Autodesk Fusion 360 part; units mm, degrees
note: some values were not read from the file. Set by a fixed rule: which sketch regions a step uses.
(part 3 of 4)
  spline S124 degree 3 poles (20.1789, 42.1401) (19.8683, 42.9655) (19.3311, 43.6836) (18.669, 44.2614) (18.1917, 44.6778) (17.6457, 45.021) (17.0294, 45.2285) knots 0.1236 0.1236 0.1236 0.1236 0.632884 0.632884 0.632884 1 1 1 1
  spline S125 degree 3 poles (17.0294, 45.2285) (15.6679, 45.6868) (14.1945, 45.6326) (12.6935, 45.1125) (12.1298, 44.9172) (11.5566, 44.6602) (10.9624, 44.3448) knots 0 0 0 0 0.726997 0.726997 0.726997 1 1 1 1
  spline S126 degree 3 poles (10.9624, 44.3448) (10.8083, 44.263) (10.6793, 44.1929) (10.573, 44.1362) knots 0 0 0 0 0.122244 0.122244 0.122244 0.122244
  spline S127 degree 3 poles (10.573, 44.1362) (10.4946, 44.2052) (10.4022, 44.2872) (10.2936, 44.382) knots 0.893888 0.893888 0.893888 0.893888 1 1 1 1
  ellipse E6 centre (-1.4228, 24.3555) end of major axis (-10.8734, 2.8827) minor radius 14.2538 (10.2936, 44.382) -> (7.2449, 46.1286) ccw
  spline S128 degree 3 poles (7.2449, 46.1286) (6.4114, 46.403) (5.4613, 46.5014) (4.5483, 46.4889) (3.8849, 46.4798) (3.2641, 46.4203) (2.6738, 46.2166) knots 0.000001 0.000001 0.000001 0.000001 0.579134 0.579134 0.579134 1 1 1 1
  spline S129 degree 3 poles (2.6737, 46.2166) (0.624, 45.5094) (-0.7902, 43.8549) (-1.106, 41.9528) (-1.287, 40.8624) (-1.1003, 39.6959) (-0.5192, 38.6497) knots 0 0 0 0 0.618555 0.618555 0.618555 0.973163 0.973163 0.973163 0.973163
  spline S130 degree 3 poles (-0.5192, 38.6497) (-0.9554, 37.9197) (-1.2418, 37.1573) (-1.2576, 36.3503) (-1.2716, 35.6348) (-1.0747, 34.9439) (-0.7598, 34.2709) knots 0.006673 0.006673 0.006673 0.006673 0.533212 0.533212 0.533212 1 1 1 1
  spline S131 degree 3 poles (-0.7598, 34.2709) (0.1145, 32.4027) (1.9335, 31.179) (4.0147, 30.9406) knots 0 0 0 0 0.893312 0.893312 0.893312 0.893312
  spline S132 degree 3 poles (4.0147, 30.9406) (3.9761, 30.3012) (3.9008, 29.105) (3.8396, 28.1591) knots 0.081568 0.081568 0.081568 0.081568 1 1 1 1
  spline S133 degree 3 poles (29.7007, 2.1311) (29.5989, 2.131) (29.4934, 2.1308) (29.3841, 2.1308) knots 0.955909 0.955909 0.955909 0.955909 1 1 1 1
  spline S134 degree 3 poles (29.3841, 2.1308) (26.2893, 2.1292) (25.7344, 2.1938) (23.1155, 2.861) knots 0 0 0 0 1 1 1 1
  spline S135 degree 3 poles (23.1155, 2.861) (15.8271, 4.7179) (10.0738, 9.8891) (7.9282, 16.5117) knots 0 0 0 0 1 1 1 1
  spline S136 degree 3 poles (7.9282, 16.5117) (7.4178, 18.087) (7.2808, 18.6726) (7.0133, 20.4204) knots 0 0 0 0 1 1 1 1
  spline S137 degree 3 poles (7.0133, 20.4204) (6.814, 21.7234) (6.7809, 22.3775) (6.7737, 25.1631) knots 0 0 0 0 1 1 1 1
  spline S138 degree 3 poles (6.7737, 25.1631) (6.7643, 28.8189) (6.9545, 31.8997) (7.2227, 32.4341) knots 0 0 0 0 1 1 1 1
  spline S139 degree 3 poles (7.2227, 32.4341) (7.3731, 32.7338) (7.7563, 33.027) (8.0031, 33.0312) knots 0 0 0 0 1 1 1 1
  spline S140 degree 3 poles (8.0031, 33.0312) (8.0532, 33.032) (8.369, 32.8492) (8.705, 32.6248) knots 0 0 0 0 1 1 1 1
  spline S141 degree 3 poles (8.705, 32.6248) (9.2851, 32.2374) (9.8665, 32.0076) (11.2214, 31.6303) knots 0 0 0 0 1 1 1 1
  spline S142 degree 3 poles (11.2214, 31.6303) (11.8742, 31.4485) (11.8914, 31.4155) (11.7143, 30.6874) knots 0 0 0 0 1 1 1 1
  spline S143 degree 3 poles (11.7143, 30.6874) (10.9845, 27.6875) (10.9096, 23.7891) (11.5242, 20.7853) knots 0 0 0 0 1 1 1 1
  spline S144 degree 3 poles (11.5242, 20.7853) (12.8947, 14.087) (17.7674, 9.0084) (23.8364, 7.9527) knots 0 0 0 0 1 1 1 1
  spline S145 degree 3 poles (23.8364, 7.9527) (24.5674, 7.8255) (25.2101, 7.7982) (26.5177, 7.8388) knots 0 0 0 0 1 1 1 1
  spline S146 degree 3 poles (26.5177, 7.8388) (26.6332, 7.8424) (26.7451, 7.8465) (26.8538, 7.8512) knots 0 0 0 0 0.059413 0.059413 0.059413 0.059413
  spline S147 degree 3 poles (26.8538, 7.8512) (26.956, 7.4679) (27.0677, 7.0952) (27.1887, 6.732) (27.7682, 4.9924) (28.5742, 3.4395) (29.7007, 2.1311) knots 0.438432 0.438432 0.438432 0.438432 0.510571 0.510571 0.510571 0.856047 0.856047 0.856047 0.856047
  spline S148 degree 3 poles (26.6696, 28.6099) (26.7348, 28.5375) (26.8011, 28.467) (26.8689, 28.3977) (27.0173, 28.2462) (27.1722, 28.1018) (27.3333, 27.9647) (27.737, 27.6213) (28.176, 27.3243) (28.6406, 27.0754) knots 0.472088 0.472088 0.472088 0.472088 0.50252 0.50252 0.50252 0.569109 0.569109 0.569109 0.739021 0.739021 0.739021 0.739021
  spline S149 degree 3 poles (28.6406, 27.0754) (28.6443, 25.9855) (28.5938, 25.3432) (28.4946, 24.805) (28.467, 24.6548) (28.4349, 24.5095) (28.3963, 24.3575) (28.3479, 24.1671) (28.2888, 23.9667) (28.2121, 23.7367) knots 0.081283 0.081283 0.081283 0.081283 0.643747 0.643747 0.643747 0.800641 0.800641 0.800641 1 1 1 1
  spline S150 degree 3 poles (28.2121, 23.7367) (27.8013, 22.5041) (27.1671, 21.814) (26.6334, 21.506) (26.5949, 21.4839) (26.5569, 21.4635) (26.5191, 21.4448) knots 0 0 0 0 0.932819 0.932819 0.932819 1 1 1 1
  spline S151 degree 3 poles (26.5191, 21.4448) (26.1495, 21.2616) (26.0295, 21.2395) (26.0131, 21.2366) (26.0049, 21.2352) (26.0092, 21.2344) (25.9705, 21.2347) (25.9474, 21.235) (25.8975, 21.2362) (25.7646, 21.2632) knots 0.000002 0.000002 0.000002 0.000002 0.475564 0.475564 0.475564 0.711303 0.711303 0.711303 1 1 1 1
  spline S152 degree 3 poles (25.7646, 21.2632) (25.182, 21.3821) (24.7581, 21.6128) (24.2876, 22.1275) (24.0894, 22.3445) (23.8887, 22.6165) (23.6933, 22.956) (23.3548, 23.5442) (23.0502, 24.3309) (22.8535, 25.2998) knots 0 0 0 0 0.460583 0.460583 0.460583 0.654705 0.654705 0.654705 1 1 1 1
  spline S153 degree 3 poles (22.8535, 25.2998) (22.8074, 25.5265) (22.7339, 26.019) (22.6741, 26.5602) knots 0 0 0 0 0.263291 0.263291 0.263291 0.263291
  spline S154 degree 3 poles (22.6741, 26.5602) (22.7213, 26.5673) (22.7686, 26.5749) (22.8158, 26.583) (23.4027, 26.6834) (23.8706, 26.8599) (24.2061, 27.0017) knots 0.562128 0.562128 0.562128 0.562128 0.599835 0.599835 0.599835 1 1 1 1
  spline S155 degree 3 poles (24.2061, 27.0017) (25.082, 27.3721) (25.9389, 27.8878) (26.6696, 28.6099) knots 0.000003 0.000003 0.000003 0.000003 0.418346 0.418346 0.418346 0.418346
  spline S156 degree 3 poles (28.691, -3.3614) (32.9408, -3.4991) (36.8407, -2.8286) (40.1448, -1.2746) knots -0.538333 -0.538333 -0.538333 -0.538333 -0.206763 -0.206763 -0.206763 -0.206763
  spline S157 degree 3 poles (40.1448, -1.2746) (41.8108, -0.4911) (43.2001, 0.4189) (44.4435, 1.5947) knots 0 0 0 0 1 1 1 1
  spline S158 degree 3 poles (44.4435, 1.5947) (46.2822, 3.3334) (47.6676, 5.4847) (48.6623, 8.151) (48.7328, 8.34) (48.8016, 8.5317) (48.8687, 8.7262) (49.3481, 10.1146) (49.753, 11.6445) (50.1382, 13.3968) knots 0 0 0 0 0.632917 0.632917 0.632917 0.677783 0.677783 0.677783 1 1 1 1
  spline S159 degree 3 poles (50.1382, 13.3968) (51.1058, 17.7988) (51.5387, 21.0845) (51.8213, 26.4015) (51.8462, 26.8705) (51.8701, 27.3558) (51.8932, 27.8597) (51.8932, 27.8597) (51.8932, 27.8597) (51.8932, 27.8597) knots 0 0 0 0 0.918938 0.918938 0.918938 1 1 1 1.000001 1.000001 1.000001 1.000001
  spline S160 degree 3 poles (51.9001, 28.0088) (51.8978, 27.959) (51.8955, 27.9093) (51.8932, 27.8597) knots 1.612217 1.612217 1.612217 1.612217 1.675112 1.675112 1.675112 1.675112
  spline S161 degree 3 poles (51.9001, 28.0088) (53.1132, 28.4408) (54.2432, 29.0437) (55.2159, 29.8879) (55.4306, 30.0742) (55.637, 30.272) (55.8334, 30.481) (56.3444, 31.0248) (56.7853, 31.6466) (57.1251, 32.3371) knots 0.244983 0.244983 0.244983 0.244983 0.667487 0.667487 0.667487 0.760746 0.760746 0.760746 0.999997 0.999997 0.999997 0.999997
  spline S162 degree 3 poles (57.1251, 32.3371) (57.3415, 32.7769) (57.5858, 33.3542) (57.7015, 34.0837) (57.7667, 34.4952) (57.7814, 34.8692) (57.7845, 35.1895) (57.7846, 35.1948) (57.7846, 35.2002) (57.7847, 35.2056) knots 0.00001 0.00001 0.00001 0.00001 0.549059 0.549059 0.549059 0.90483 0.90483 0.90483 0.912062 0.912062 0.912062 0.912062
  line L17 (57.7847, 35.2056) -> (57.7832, 35.6708)
  spline S163 degree 3 poles (57.7832, 35.6708) (57.7831, 35.6767) (57.783, 35.6826) (57.7829, 35.6885) (57.7753, 36.1231) (57.7439, 36.6405) (57.6135, 37.201) (57.5259, 37.5777) (57.4101, 37.9108) (57.2954, 38.2005) knots 0.081345 0.081345 0.081345 0.081345 0.088946 0.088946 0.088946 0.543269 0.543269 0.543269 0.85612 0.85612 0.85612 0.85612
  spline S164 degree 3 poles (57.2954, 38.2005) (57.6289, 40.0462) (57.2005, 41.9011) (56.2368, 43.3879) (56.0215, 43.7199) (55.7793, 44.0349) (55.5119, 44.3297) (54.486, 45.4604) (53.1277, 46.2732) (51.6026, 46.6806) knots 0.058405 0.058405 0.058405 0.058405 0.508016 0.508016 0.508016 0.608426 0.608426 0.608426 1 1 1 1
  spline S165 degree 3 poles (51.6026, 46.6806) (50.3461, 47.0162) (49.0649, 46.9995) (47.8164, 46.7767) knots 0.000001 0.000001 0.000001 0.000001 0.638334 0.638334 0.638334 0.638334
  spline S166 degree 3 poles (47.8164, 46.7767) (47.5813, 47.0383) (47.3201, 47.2937) (47.0295, 47.534) (46.9498, 47.5999) (46.864, 47.6675) (46.7723, 47.7352) knots 0.700865 0.700865 0.700865 0.700865 0.939053 0.939053 0.939053 0.999998 0.999998 0.999998 0.999998
  spline S167 degree 3 poles (46.7723, 47.7352) (45.3302, 48.7994) (43.6443, 49.2146) (42.0523, 49.2386) (41.9141, 49.2407) (41.7762, 49.2398) (41.6389, 49.2361) (40.9851, 49.2182) (40.3133, 49.1301) (39.6411, 48.9493) knots 0.000002 0.000002 0.000002 0.000002 0.67158 0.67158 0.67158 0.729882 0.729882 0.729882 1 1 1 1
  spline S168 degree 3 poles (39.6411, 48.9493) (38.4909, 48.64) (37.4459, 48.1024) (36.5017, 47.4327) knots 0.000003 0.000003 0.000003 0.000003 0.699439 0.699439 0.699439 0.699439
  spline S169 degree 3 poles (36.5017, 47.4327) (34.5065, 48.0801) (32.3383, 47.9768) (30.4458, 47.0772) (28.9141, 46.3491) (27.639, 45.1486) (26.7459, 43.6578) knots 0.150615 0.150615 0.150615 0.150615 0.618328 0.618328 0.618328 1 1 1 1
  spline S170 degree 3 poles (26.7459, 43.6578) (26.4916, 43.2334) (26.2811, 42.7867) (26.1168, 42.3268) knots 0 0 0 0 0.168016 0.168016 0.168016 0.168016
  spline S171 degree 3 poles (26.1168, 42.3268) (25.625, 42.8719) (25.0259, 43.3578) (24.3244, 43.7251) (23.4812, 44.1666) (22.6044, 44.3989) (21.7478, 44.5189) knots 0.247509 0.247509 0.247509 0.247509 0.510228 0.510228 0.510228 0.845044 0.845044 0.845044 0.845044
  spline S172 degree 3 poles (21.7478, 44.5189) (21.336, 45.137) (20.8474, 45.6785) (20.3127, 46.145) (19.6364, 46.7352) (18.8102, 47.2669) (17.827, 47.5978) knots 0.340303 0.340303 0.340303 0.340303 0.632884 0.632884 0.632884 1 1 1 1
  spline S173 degree 3 poles (17.827, 47.5978) (15.8921, 48.2491) (13.8035, 48.1429) (11.8751, 47.4748) (11.5408, 47.359) (11.2106, 47.2283) (10.8834, 47.0845) knots 0 0 0 0 0.726997 0.726997 0.726997 0.855649 0.855649 0.855649 0.855649
  spline S174 degree 3 poles (10.8834, 47.0845) (10.0021, 47.6912) (9.04, 48.1696) (8.0266, 48.5032) knots 3.02631 3.02631 3.02631 3.02631 3.200385 3.200385 3.200385 3.200385
  spline S175 degree 3 poles (8.0266, 48.5032) (6.8258, 48.8985) (5.6304, 49.004) (4.514, 48.9887) (3.7224, 48.9778) (2.8175, 48.9108) (1.8584, 48.5799) knots 0.000001 0.000001 0.000001 0.000001 0.579134 0.579134 0.579134 1 1 1 1
  spline S176 degree 3 poles (1.8584, 48.5799) (-0.9926, 47.5963) (-3.0973, 45.223) (-3.5722, 42.3622) (-3.7722, 41.1577) (-3.6732, 39.9046) (-3.2719, 38.717) knots 0 0 0 0 0.618555 0.618555 0.618555 0.877662 0.877662 0.877662 0.877662
  spline S177 degree 3 poles (-3.2719, 38.717) (-3.5504, 38.0202) (-3.7407, 37.2387) (-3.7571, 36.3992) (-3.7807, 35.1938) (-3.4479, 34.1169) (-3.0241, 33.2113) knots 0.209942 0.209942 0.209942 0.209942 0.533212 0.533212 0.533212 1 1 1 1
  spline S178 degree 3 poles (-3.0241, 33.2113) (-2.118, 31.2751) (-0.5085, 29.8275) (1.3919, 29.0531) knots 0 0 0 0 0.64194 0.64194 0.64194 0.64194
  spline S179 degree 3 poles (1.3919, 29.0531) (1.3758, 28.8015) (1.3599, 28.5533) (1.3448, 28.3205) knots 0.773012 0.773012 0.773012 0.773012 1 1 1 1
  spline S180 degree 3 poles (1.3448, 28.3205) (1.1855, 25.8574) (1.2497, 22.768) (1.5259, 20.4573) knots 0 0 0 0 1 1 1 1
  spline S181 degree 3 poles (1.5259, 20.4573) (2.188, 14.9161) (4.3341, 9.9177) (7.8149, 5.9804) (8.3213, 5.4077) (8.8549, 4.8572) (9.4145, 4.3301) knots 2.814804 2.814804 2.814804 2.814804 3.195269 3.195269 3.195269 3.250613 3.250613 3.250613 3.250613
  spline S182 degree 3 poles (9.4145, 4.3301) (14.1533, -0.1335) (20.1834, -2.7036) (26.9457, -3.2616) (27.5221, -3.3091) (28.1039, -3.3424) (28.691, -3.3614) (28.691, -3.3614) (28.691, -3.3614) (28.691, -3.3614) knots 0 0 0 0 0.921454 0.921454 0.921454 1 1 1 1.000001 1.000001 1.000001 1.000001
  spline S183 degree 3 poles (28.8529, 1.636) (32.482, 1.5184) (35.5808, 2.1042) (38.0169, 3.25) knots -0.538331 -0.538331 -0.538331 -0.538331 -0.206759 -0.206759 -0.206759 -0.206759
  spline S184 degree 3 poles (38.0169, 3.25) (38.0169, 3.25) (38.0169, 3.25) (38.0169, 3.25) (39.3378, 3.8712) (40.1452, 4.4117) (41.0081, 5.2276) knots -0.000007 -0.000007 -0.000007 -0.000007 0 0 0 1 1 1 1
  spline S185 degree 3 poles (41.0081, 5.2276) (42.2991, 6.4485) (43.1918, 7.792) (43.9777, 9.8986) (44.0334, 10.048) (44.0883, 10.2011) (44.1425, 10.358) (44.5347, 11.4938) (44.8968, 12.8414) (45.2548, 14.4702) knots 0 0 0 0 0.632917 0.632917 0.632917 0.677783 0.677783 0.677783 1 1 1 1
  spline S186 degree 3 poles (45.2548, 14.4702) (46.1799, 18.6789) (46.5538, 21.5025) (46.8283, 26.6668) (46.8525, 27.1224) (46.8758, 27.5957) (46.8985, 28.0892) knots 0 0 0 0 0.918938 0.918938 0.918938 1 1 1 1
  spline S187 degree 3 poles (47.4971, 32.0539) (47.4947, 32.0505) (47.4924, 32.0471) (47.4902, 32.0437) (47.2657, 31.7128) (47.2344, 31.5681) (47.1957, 31.4563) (47.1118, 31.2144) (47.1097, 31.1501) (47.0977, 31.0856) (47.0666, 30.9194) (47.0663, 30.88) (47.06, 30.8195) (47.0394, 30.6238) (47.0264, 30.4292) (47.0081, 30.1441) (46.974, 29.6114) (46.9329, 28.8378) (46.8985, 28.0892) knots 0.02505 0.02505 0.02505 0.02505 0.025328 0.025328 0.025328 0.052584 0.052584 0.052584 0.111532 0.111532 0.111532 0.263489 0.263489 0.263489 0.755669 0.755669 0.755669 1.675088 1.675088 1.675088 1.675088
  spline S188 degree 3 poles (47.4971, 32.0539) (47.9897, 32.1595) (48.4824, 32.2652) (48.975, 32.3709) (50.3458, 32.665) (51.3246, 33.1312) (51.9386, 33.6641) (52.029, 33.7425) (52.1123, 33.8226) (52.1898, 33.9051) (52.3815, 34.1091) (52.5305, 34.3245) (52.6389, 34.5448) knots -0.155756 -0.155756 -0.155756 -0.155756 0.033409 0.033409 0.033409 0.667487 0.667487 0.667487 0.760746 0.760746 0.760746 0.999995 0.999995 0.999995 0.999995
  spline S189 degree 3 poles (52.6389, 34.5448) (52.6389, 34.5448) (52.6389, 34.5448) (52.6389, 34.5448) (52.7279, 34.7256) (52.7597, 34.8448) (52.7632, 34.8668) (52.7748, 34.9403) (52.7824, 35.0261) (52.7846, 35.2226) knots -0.000017 -0.000017 -0.000017 -0.000017 0 0 0 0.549059 0.549059 0.549059 0.896086 0.896086 0.896086 0.896086
  line L18 (52.7846, 35.2226) -> (52.7833, 35.6181)
  spline S190 degree 3 poles (52.7833, 35.6181) (52.7783, 35.8758) (52.7642, 35.9794) (52.7436, 36.0679) (52.7193, 36.1724) (52.6747, 36.3015) (52.5459, 36.602) knots 0.098297 0.098297 0.098297 0.098297 0.543269 0.543269 0.543269 1 1 1 1
  line L19 (52.5459, 36.602) -> (52.0202, 37.8281)
  line L20 (52.0202, 37.8281) -> (52.325, 38.8768)
  spline S191 degree 3 poles (52.325, 38.8768) (52.5054, 39.4971) (52.39, 40.1301) (52.0412, 40.6681) (51.9722, 40.7745) (51.8944, 40.8757) (51.8089, 40.97) (51.4582, 41.3565) (50.9527, 41.6789) (50.3122, 41.8499) knots 0.000001 0.000001 0.000001 0.000001 0.508016 0.508016 0.508016 0.608426 0.608426 0.608426 1 1 1 1
  spline S192 degree 3 poles (50.3122, 41.8499) (49.8357, 41.9772) (49.2359, 41.9882) (48.3226, 41.7781) (48.2236, 41.7553) (48.1214, 41.73) (48.016, 41.702) (47.8566, 41.6597) (47.6893, 41.6113) (47.5135, 41.5566) (46.8495, 41.3501) (46.1854, 41.1435) (45.5213, 40.937) knots 0 0 0 0 0.74388 0.74388 0.74388 0.824545 0.824545 0.824545 0.945665 0.945665 0.945665 1.335942 1.335942 1.335942 1.335942
  spline S193 degree 3 poles (45.5213, 40.937) (45.1993, 41.5534) (44.8773, 42.1698) (44.5552, 42.7862) (44.5311, 42.8323) (44.4975, 42.8908) (44.4575, 42.9537) (44.2603, 43.2641) (44.0459, 43.5132) (43.8431, 43.6809) (43.827, 43.6942) (43.8143, 43.704) (43.8035, 43.712) knots -0.495914 -0.495914 -0.495914 -0.495914 0.223295 0.223295 0.223295 0.361232 0.361232 0.361232 0.939053 0.939053 0.939053 1 1 1 1
  spline S194 degree 3 poles (43.8035, 43.712) (43.3808, 44.0239) (42.7445, 44.2276) (41.9768, 44.2392) (41.9102, 44.2402) (41.8429, 44.2398) (41.7751, 44.2379) (41.4784, 44.2298) (41.1969, 44.1901) (40.9398, 44.1209) knots 0.000002 0.000002 0.000002 0.000002 0.67158 0.67158 0.67158 0.729882 0.729882 0.729882 1 1 1 1
  spline S195 degree 3 poles (40.9397, 44.1209) (40.2839, 43.9445) (39.4481, 43.4741) (38.7124, 42.8035) knots 0.000001 0.000001 0.000001 0.000001 1 1 1 1
  line L21 (38.7124, 42.8035) -> (37.2495, 41.4699)
  spline S196 degree 3 poles (37.2495, 41.4699) (36.724, 41.767) (36.1986, 42.0641) (35.6731, 42.3611) (34.5938, 42.9714) (33.4845, 42.9855) (32.5924, 42.5614) (32.0115, 42.2853) (31.4617, 41.8003) (31.0351, 41.0882) knots -0.162297 -0.162297 -0.162297 -0.162297 0.019099 0.019099 0.019099 0.618328 0.618328 0.618328 1 1 1 1
  spline S197 degree 3 poles (31.0351, 41.0882) (30.7054, 40.5379) (30.5949, 39.9065) (30.737, 39.2208) (30.822, 38.8109) (30.9944, 38.3422) (31.2817, 37.8012) knots 0 0 0 0 0.647645 0.647645 0.647645 1 1 1 1
  line L22 (31.2817, 37.8012) -> (32.2313, 36.013)
  line L23 (32.2313, 36.013) -> (30.7684, 34.5336)
  spline S198 degree 3 poles (30.7684, 34.5336) (30.3425, 34.1029) (30.1555, 33.8199) (30.0718, 33.6163) (30.063, 33.595) (30.0551, 33.5742) (30.0479, 33.5532) (30.0006, 33.4158) (29.9666, 33.22) (29.9688, 32.9384) knots 0 0 0 0 0.54646 0.54646 0.54646 0.603605 0.603605 0.603605 1 1 1 1
  spline S199 degree 3 poles (29.9688, 32.9384) (29.9715, 32.5856) (30.1268, 32.2171) (30.4414, 31.8959) (30.4831, 31.8533) (30.5271, 31.8122) (30.5732, 31.7731) (30.8562, 31.5323) (31.2343, 31.3328) (31.6987, 31.2194) (32.2182, 31.0926) (32.7376, 30.9658) (33.2571, 30.839) knots 0 0 0 0 0.50252 0.50252 0.50252 0.569109 0.569109 0.569109 0.954182 0.954182 0.954182 1.198713 1.198713 1.198713 1.198713
  spline S200 degree 3 poles (33.6349, 27.6578) (33.6265, 28.1881) (33.6121, 28.719) (33.5943, 29.1314) (33.5834, 29.3845) (33.5734, 29.5797) (33.5545, 29.7812) (33.5487, 29.8427) (33.5428, 29.9038) (33.5287, 29.9983) (33.5177, 30.0719) (33.5151, 30.1431) (33.445, 30.3784) (33.4163, 30.4747) (33.3945, 30.5926) (33.2571, 30.839) knots -1.60234 -1.60234 -1.60234 -1.60234 -0.832399 -0.832399 -0.832399 -0.359926 -0.359926 -0.359926 -0.215638 -0.215638 -0.215638 -0.103142 -0.103142 -0.103142 -0.0571 -0.0571 -0.0571 -0.0571
  spline S201 degree 3 poles (33.6349, 27.6578) (33.6595, 26.1101) (33.6111, 24.9803) (33.4119, 23.899) (33.3633, 23.6355) (33.3064, 23.3782) (33.2423, 23.126) (33.1601, 22.8028) (33.0643, 22.4819) (32.9556, 22.1557) knots 0.000004 0.000004 0.000004 0.000004 0.643747 0.643747 0.643747 0.800641 0.800641 0.800641 1 1 1 1
  spline S202 degree 3 poles (32.9556, 22.1557) (32.2317, 19.9839) (30.9202, 18.2069) (29.1322, 17.1752) (29.0034, 17.1009) (28.8723, 17.0307) (28.7391, 16.9647) knots 0 0 0 0 0.932819 0.932819 0.932819 1 1 1 1
  spline S203 degree 3 poles (28.7391, 16.9647) (28.1265, 16.6611) (27.5201, 16.4228) (26.8636, 16.3095) (26.5381, 16.2533) (26.2135, 16.2321) (25.9203, 16.235) (25.5368, 16.2389) (25.1482, 16.286) (24.7656, 16.3641) knots 0 0 0 0 0.475564 0.475564 0.475564 0.711303 0.711303 0.711303 1 1 1 1
  spline S204 degree 3 poles (24.7656, 16.3641) (23.1787, 16.6877) (21.7086, 17.538) (20.5969, 18.7544) (20.1283, 19.2671) (19.7176, 19.8402) (19.3597, 20.4621) (18.714, 21.584) (18.2438, 22.8744) (17.9534, 24.3051) knots 0 0 0 0 0.460583 0.460583 0.460583 0.654705 0.654705 0.654705 1 1 1 1
  spline S205 degree 3 poles (17.9534, 24.3051) (17.831, 24.9081) (17.7431, 25.6067) (17.667, 26.3655) (17.6316, 26.7176) (17.6007, 27.0766) (17.5759, 27.4273) (17.5378, 27.9642) (17.5129, 28.4767) (17.5049, 28.924) (17.4937, 29.549) (17.4825, 30.174) (17.4713, 30.7991) knots 0 0 0 0 0.312333 0.312333 0.312333 0.457255 0.457255 0.457255 0.680586 0.680586 0.680586 1.042282 1.042282 1.042282 1.042282
  spline S206 degree 3 poles (20.5802, 31.4721) (20.0763, 31.4736) (19.6513, 31.4671) (19.2861, 31.444) (19.1179, 31.4334) (18.9789, 31.4265) (18.7326, 31.3824) (18.6233, 31.3629) (18.5023, 31.3481) (18.2322, 31.2466) (18.1014, 31.1975) (17.9317, 31.1353) (17.6625, 30.947) (17.6036, 30.9057) (17.5377, 30.858) (17.4713, 30.7991) knots 2.063963 2.063963 2.063963 2.063963 2.635195 2.635195 2.635195 2.89832 2.89832 2.89832 3.015054 3.015054 3.015054 3.071597 3.071597 3.071597 3.08397 3.08397 3.08397 3.08397
  spline S207 degree 3 poles (20.5802, 31.4721) (21.2817, 31.47) (21.6536, 31.4748) (21.8409, 31.4937) (21.891, 31.4987) (21.9311, 31.5042) (21.9723, 31.5113) (22.0174, 31.519) (22.1165, 31.5468) (22.259, 31.6071) (22.259, 31.6071) (22.259, 31.6071) (22.2591, 31.6071) knots 0 0 0 0 0.47317 0.47317 0.47317 0.599835 0.599835 0.599835 1 1 1 1.00001 1.00001 1.00001 1.00001
  spline S208 degree 3 poles (22.2591, 31.6071) (22.8153, 31.8423) (23.1441, 32.116) (23.3079, 32.3433) (23.3351, 32.381) (23.3587, 32.4182) (23.3798, 32.4562) (23.4541, 32.5898) (23.5115, 32.7711) (23.5276, 32.9724) knots 0.000003 0.000003 0.000003 0.000003 0.559796 0.559796 0.559796 0.65253 0.65253 0.65253 1 1 1 1
  spline S209 degree 3 poles (23.5276, 32.9724) (23.5484, 33.2315) (23.5378, 33.2897) (23.536, 33.2991) (23.5329, 33.3147) (23.5221, 33.3646) (23.4326, 33.5601) (23.4326, 33.5601) (23.4326, 33.5602) (23.4326, 33.5602) knots 0 0 0 0 0.532706 0.532706 0.532706 1 1 1 1.00001 1.00001 1.00001 1.00001
  spline S210 degree 3 poles (23.4326, 33.5602) (23.2318, 33.9987) (22.7513, 34.604) (21.9766, 35.1834) knots 0.355118 0.355118 0.355118 0.355118 0.81789 0.81789 0.81789 0.81789
  spline S211 degree 3 poles (21.9766, 35.1834) (22.2344, 35.7237) (22.4922, 36.2639) (22.75, 36.8042) (22.821, 36.9529) (22.8776, 37.1492) (22.8965, 37.372) (22.9021, 37.4387) (22.907, 37.5155) (22.9112, 37.6065) knots -0.861715 -0.861715 -0.861715 -0.861715 0.077995 0.077995 0.077995 0.83962 0.83962 0.83962 1 1 1 1
  spline S212 degree 3 poles (22.9112, 37.6065) (22.9267, 37.9446) (22.9226, 38.029) (22.9163, 38.0717) (22.9157, 38.076) (22.915, 38.0803) (22.9141, 38.0851) knots 0 0 0 0 0.440308 0.440308 0.440308 0.484514 0.484514 0.484514 0.484514
  spline S213 degree 3 poles (22.9141, 38.0851) (22.9136, 38.0875) (22.9006, 38.1464) (22.8052, 38.3453) (22.7894, 38.3781) (22.7719, 38.414) (22.7524, 38.4537) knots 0.500669 0.500669 0.500669 0.500669 0.930484 0.930484 0.930484 1 1 1 1
  spline S214 degree 3 poles (22.7524, 38.4537) (22.5414, 38.8823) (22.2676, 39.1581) (22.0052, 39.2955) (21.7005, 39.455) (21.2598, 39.5735) (20.5069, 39.6207) (20.4537, 39.6241) (20.3992, 39.627) (20.3434, 39.6297) knots 0 0 0 0 0.510228 0.510228 0.510228 0.967706 0.967706 0.967706 1 1 1 1
  line L24 (20.3434, 39.6297) -> (18.4188, 39.7197)
  spline S215 degree 3 poles (18.4188, 39.7197) (18.2256, 40.2329) (18.0324, 40.7461) (17.8392, 41.2593) (17.6948, 41.643) (17.4188, 42.0343) (17.0253, 42.3777) (16.7471, 42.6205) (16.4812, 42.7752) (16.2319, 42.8591) knots -0.193067 -0.193067 -0.193067 -0.193067 0.1236 0.1236 0.1236 0.632884 0.632884 0.632884 1 1 1 1
  spline S216 degree 3 poles (16.2319, 42.8591) (15.4436, 43.1244) (14.5856, 43.1223) (13.5119, 42.7503) (13.0939, 42.6055) (12.6374, 42.4036) (12.1347, 42.1367) knots 0 0 0 0 0.726997 0.726997 0.726997 1 1 1 1
  spline S217 degree 3 poles (12.1347, 42.1367) (11.9925, 42.0612) (11.8697, 41.9944) (11.7497, 41.9304) (11.2403, 41.6587) (10.731, 41.387) (10.2217, 41.1153) knots 0 0 0 0 0.122244 0.122244 0.122244 0.708101 0.708101 0.708101 0.708101
  spline S218 degree 3 poles (10.2217, 41.1153) (9.7883, 41.4966) (9.3549, 41.878) (8.9216, 42.2593) (8.8359, 42.3347) (8.749, 42.4119) (8.6504, 42.4979) knots 0.307309 0.307309 0.307309 0.307309 0.893888 0.893888 0.893888 1 1 1 1
  spline S219 degree 3 poles (8.6504, 42.4979) (7.9831, 43.0799) (7.2588, 43.492) (6.4631, 43.754) knots 2.954129 2.954129 2.954129 2.954129 3.200387 3.200387 3.200387 3.200387
  spline S220 degree 3 poles (6.4631, 43.754) (5.9969, 43.9074) (5.2921, 43.9989) (4.5826, 43.9891) (4.0473, 43.9818) (3.7108, 43.9298) (3.4891, 43.8533) knots 0.000001 0.000001 0.000001 0.000001 0.579134 0.579134 0.579134 1 1 1 1
  spline S221 degree 3 poles (3.4891, 43.8533) (2.2407, 43.4226) (1.5169, 42.4869) (1.3603, 41.5434) (1.2719, 41.011) (1.3578, 40.4189) (1.6662, 39.8637) (1.8994, 39.4439) (2.1326, 39.0241) (2.3658, 38.6043) knots 0.000001 0.000001 0.000001 0.000001 0.618555 0.618555 0.618555 0.973163 0.973163 0.973163 1.115459 1.115459 1.115459 1.115459
  spline S222 degree 3 poles (2.3658, 38.6043) (2.1195, 38.1921) (1.8732, 37.7798) (1.6269, 37.3676) (1.3366, 36.8816) (1.2467, 36.548) (1.2419, 36.3014) (1.2375, 36.0758) (1.2985, 35.771) (1.5046, 35.3306) knots -0.290647 -0.290647 -0.290647 -0.290647 0.006673 0.006673 0.006673 0.533212 0.533212 0.533212 1 1 1 1
  spline S223 degree 3 poles (1.5046, 35.3306) (1.9464, 34.3864) (2.8224, 33.7143) (3.9435, 33.4815) (4.0598, 33.4573) (4.1785, 33.4382) (4.2992, 33.4244) (5.0838, 33.3345) (5.8684, 33.2446) (6.653, 33.1547) knots 0 0 0 0 0.809326 0.809326 0.809326 0.893312 0.893312 0.893312 1.230091 1.230091 1.230091 1.230091
  spline S224 degree 3 poles (6.653, 33.1547) (6.6054, 32.3665) (6.5578, 31.5782) (6.5101, 30.7899) (6.471, 30.1427) (6.3958, 28.9474) (6.3344, 27.9977) knots -1.050718 -1.050718 -1.050718 -1.050718 0.081568 0.081568 0.081568 1 1 1 1
  spline S225 degree 3 poles (6.3344, 27.9977) (6.2001, 25.9217) (6.2704, 22.8924) (6.4905, 21.0506) knots 0 0 0 0 1 1 1 1
  spline S226 degree 3 poles (6.4905, 21.0506) (7.1275, 15.7208) (9.3016, 11.3051) (12.8428, 7.9698) knots 2.814805 2.814805 2.814805 2.814805 3.250616 3.250616 3.250616 3.250616
  spline S227 degree 3 poles (12.8428, 7.9698) (12.8428, 7.9698) (12.8428, 7.9698) (12.8428, 7.9698) (16.7533, 4.2864) (21.585, 2.1977) (27.3568, 1.7215) (27.8488, 1.6809) (28.3475, 1.6523) (28.8529, 1.636) knots -0.000002 -0.000002 -0.000002 -0.000002 0 0 0 0.921454 0.921454 0.921454 1 1 1 1
  dimension "d24" = 2.5
  dimension "d25" = -2.5
sketch "Sketch4" plane through (0, 0, -2) normal (0, 0, -1) x (1, 0, 0)
  spline S0 degree 3 poles (26.0631, 15.8423) (26.0024, 13.4447) (26.1457, 11.3703) (26.4797, 9.5307) knots 0.017136 0.017136 0.017136 0.017136 0.337125 0.337125 0.337125 0.337125
  spline S1 degree 3 poles (26.4797, 9.5307) (25.4741, 9.5023) (24.427, 9.5799) (23.6217, 9.7658) knots 0.450431 0.450431 0.450431 0.450431 1 1 1 1
  spline S2 degree 3 poles (23.6217, 9.7658) (21.0994, 10.3485) (19.0072, 11.5487) (17.1769, 13.463) knots 0 0 0 0 1 1 1 1
  spline S3 degree 3 poles (17.1769, 13.463) (13.6018, 17.2023) (12.102, 22.8928) (13.1278, 28.8262) knots 0 0 0 0 1 1 1 1
  spline S4 degree 3 poles (13.1278, 28.8262) (13.3528, 30.1278) (13.671, 31.4351) (13.8593, 31.832) knots 0 0 0 0 1 1 1 1
  spline S5 degree 3 poles (13.8593, 31.832) (14.0085, 32.1465) (14.374, 32.4073) (14.6654, 32.4073) knots 0 0 0 0 1 1 1 1
  spline S6 degree 3 poles (14.6654, 32.4073) (14.734, 32.4073) (15.313, 32.0502) (15.9519, 31.6138) knots 0 0 0 0 1 1 1 1
  line L0 (15.9519, 31.6138) -> (17.1137, 30.8202)
  line L1 (17.1137, 30.8202) -> (17.1634, 28.2522)
  spline S7 degree 3 poles (17.1634, 28.2522) (17.2317, 24.7162) (17.5594, 23.0905) (18.6473, 20.8895) knots 0 0 0 0 1 1 1 1
  spline S8 degree 3 poles (18.6473, 20.8895) (19.9291, 18.2961) (21.9531, 16.557) (24.3463, 15.9928) knots 0 0 0 0 1 1 1 1
  spline S9 degree 3 poles (24.3463, 15.9928) (24.7994, 15.886) (25.4418, 15.8358) (26.0631, 15.8423) knots 0 0 0 0 0.531523 0.531523 0.531523 0.531523
  spline S10 degree 5 poles (28.8667, 8.0774) (28.9794, 7.6798) (29.2738, 6.7511) (29.8256, 5.3923) (30.5166, 4.1992) (31.3732, 3.1762) (32.107, 2.5202) (32.4991, 2.2173) knots 0.458614 0.458614 0.458614 0.458614 0.458614 0.458614 0.6 0.8 1 1 1 1 1 1
  spline S11 degree 3 poles (28.8667, 8.0774) (29.5627, 8.226) (30.2228, 8.4596) (31.078, 8.8283) knots 0.493372 0.493372 0.493372 0.493372 1 1 1 1
  spline S12 degree 3 poles (31.078, 8.8283) (35.3425, 10.6668) (38.7599, 15.2726) (39.9599, 20.7989) knots 0 0 0 0 1 1 1 1
  spline S13 degree 3 poles (39.9599, 20.7989) (40.381, 22.7381) (40.5138, 24.5489) (40.4444, 27.4041) knots 0 0 0 0 1 1 1 1
  spline S14 degree 3 poles (40.4444, 27.4041) (40.4089, 28.866) (40.3511, 30.4904) (40.316, 31.014) knots 0 0 0 0 1 1 1 1
  line L2 (40.316, 31.014) -> (40.2522, 31.966)
  line L3 (40.2522, 31.966) -> (41.7662, 32.4472)
  spline S15 degree 3 poles (41.7662, 32.4472) (42.5989, 32.7119) (43.3335, 32.9285) (43.3985, 32.9285) knots 0 0 0 0 1 1 1 1
  spline S16 degree 3 poles (43.3985, 32.9285) (43.4636, 32.9285) (43.808, 32.6862) (44.1638, 32.39) knots 0 0 0 0 1 1 1 1
  spline S17 degree 3 poles (44.1638, 32.39) (44.5196, 32.0939) (45.2044, 31.6627) (45.6856, 31.4317) knots 0 0 0 0 1 1 1 1
  line L4 (45.6856, 31.4317) -> (46.5605, 31.0119)
  line L5 (46.5605, 31.0119) -> (46.4885, 28.8171)
  spline S18 degree 3 poles (46.4885, 28.8171) (46.2828, 22.5508) (45.6972, 17.9425) (44.4939, 13.1206) knots 0 0 0 0 1 1 1 1
  spline S19 degree 3 poles (44.4939, 13.1206) (43.6086, 9.573) (42.6843, 7.6473) (41.0419, 5.9282) knots 0 0 0 0 1 1 1 1
  spline S20 degree 3 poles (41.0419, 5.9282) (39.2602, 4.0633) (36.9993, 2.991) (33.5472, 2.3735) knots 0 0 0 0 1 1 1 1
  spline S21 degree 3 poles (33.5472, 2.3735) (33.1543, 2.3032) (32.8372, 2.253) (32.4991, 2.2173) knots 0 0 0 0 0.330606 0.330606 0.330606 0.330606
  spline S22 degree 3 poles (28.0734, 16.1624) (30.4154, 16.9952) (32.4795, 19.2422) (33.3899, 22.0071) knots 0.073406 0.073406 0.073406 0.073406 1 1 1 1
  spline S23 degree 3 poles (33.3899, 22.0071) (33.9317, 23.6526) (34.039, 24.4827) (34.0972, 27.4794) knots 0 0 0 0 1 1 1 1
  line L6 (34.0972, 27.4794) -> (34.1523, 30.317)
  line L7 (34.1523, 30.317) -> (34.6867, 30.7314)
  spline S24 degree 3 poles (34.6867, 30.7314) (34.9807, 30.9594) (35.5718, 31.5) (36.0003, 31.9329) knots 0 0 0 0 1 1 1 1
  spline S25 degree 3 poles (36.0003, 31.9329) (36.4288, 32.3658) (36.7897, 32.72) (36.8022, 32.72) knots 0 0 0 0 1 1 1 1
  spline S26 degree 3 poles (36.8022, 32.72) (36.8147, 32.72) (37.1676, 32.5951) (37.5865, 32.4424) knots 0 0 0 0 1 1 1 1
  spline S27 degree 3 poles (37.5865, 32.4424) (38.0054, 32.2897) (38.358, 32.1588) (38.3699, 32.1514) knots 0 0 0 0 1 1 1 1
  spline S28 degree 3 poles (38.3699, 32.1514) (38.3819, 32.1441) (38.4663, 31.4364) (38.5576, 30.5789) knots 0 0 0 0 1 1 1 1
  spline S29 degree 3 poles (38.5576, 30.5789) (38.7576, 28.7005) (38.787, 24.9492) (38.613, 23.4953) knots 0 0 0 0 1 1 1 1
  spline S30 degree 3 poles (38.613, 23.4953) (38.0797, 19.0373) (36.5859, 15.601) (34.0858, 13.0806) knots 0 0 0 0 1 1 1 1
  spline S31 degree 3 poles (34.0858, 13.0806) (32.465, 11.4468) (30.6163, 10.3222) (28.7127, 9.8123) knots 0 0 0 0 1 1 1 1
  spline S32 degree 3 poles (28.7127, 9.8123) (28.6362, 9.7918) (28.5569, 9.7724) (28.475, 9.7541) knots 0 0 0 0 0.056248 0.056248 0.056248 0.056248
  spline S33 degree 5 poles (28.0734, 16.1624) (28.0438, 15.2899) (28.0325, 13.8524) (28.0901, 12.5348) (28.2108, 11.3251) (28.3896, 10.2086) (28.475, 9.7541) knots 0 0 0 0 0 0 0.2 0.345499 0.345499 0.345499 0.345499 0.345499 0.345499
  spline S34 degree 3 poles (3.3605, 43.321) (4.2972, 43.7123) (5.127, 43.7031) (6.3837, 43.2874) knots 0 0 0 0 1 1 1 1
  spline S35 degree 3 poles (6.3837, 43.2874) (7.3845, 42.9564) (8.1509, 42.4223) (9.1149, 41.384) knots 0 0 0 0 1 1 1 1
  spline S36 degree 3 poles (9.1149, 41.384) (9.6604, 40.7965) (9.9744, 40.5375) (10.1414, 40.5375) knots 0 0 0 0 1 1 1 1
  spline S37 degree 3 poles (10.1414, 40.5375) (10.2736, 40.5375) (10.8079, 40.801) (11.3285, 41.1231) knots 0 0 0 0 1 1 1 1
  spline S38 degree 3 poles (11.3285, 41.1231) (12.8148, 42.0424) (13.5925, 42.3956) (14.4099, 42.5224) knots 0 0 0 0 1 1 1 1
  spline S39 degree 3 poles (14.4099, 42.5224) (15.7434, 42.7294) (16.8719, 42.2963) (17.2889, 41.4175) knots 0 0 0 0 1 1 1 1
  spline S40 degree 3 poles (17.2889, 41.4175) (17.4425, 41.0937) (17.464, 40.8751) (17.4081, 40.2046) knots 0 0 0 0 1 1 1 1
  spline S41 degree 3 poles (17.4081, 40.2046) (17.3434, 39.4284) (17.3531, 39.3735) (17.5983, 39.1282) knots 0 0 0 0 1 1 1 1
  spline S42 degree 3 poles (17.5983, 39.1282) (17.8995, 38.827) (18.0838, 38.8152) (19.1861, 39.0261) knots 0 0 0 0 1 1 1 1
  spline S43 degree 3 poles (19.1861, 39.0261) (21.2987, 39.4304) (22.4511, 38.9297) (22.4522, 37.607) knots 0 0 0 0 1 1 1 1
  spline S44 degree 3 poles (22.4522, 37.607) (22.4529, 36.7454) (21.8377, 36.2639) (20.7361, 36.2639) knots 0 0 0 0 1 1 1 1
  spline S45 degree 3 poles (20.7361, 36.2639) (20.0382, 36.2639) (19.7425, 36.0347) (19.7425, 35.4937) knots 0 0 0 0 1 1 1 1
  spline S46 degree 3 poles (19.7425, 35.4937) (19.7425, 34.9001) (19.9962, 34.7075) (21.0588, 34.4943) knots 0 0 0 0 1 1 1 1
  spline S47 degree 3 poles (21.0588, 34.4943) (22.1331, 34.2788) (22.5478, 34.0955) (22.8603, 33.6982) knots 0 0 0 0 1 1 1 1
  spline S48 degree 3 poles (22.8603, 33.6982) (23.5958, 32.7632) (22.5543, 31.8861) (20.7083, 31.8861) knots 0 0 0 0 1 1 1 1
  spline S49 degree 3 poles (20.7083, 31.8861) (18.9346, 31.8861) (17.432, 32.5128) (15.9552, 33.8684) knots 0 0 0 0 1 1 1 1
  spline S50 degree 3 poles (15.9552, 33.8684) (15.4567, 34.326) (14.9608, 34.7004) (14.8533, 34.7004) knots 0 0 0 0 1 1 1 1
  spline S51 degree 3 poles (14.8533, 34.7004) (14.7458, 34.7004) (14.4299, 34.5351) (14.1513, 34.333) knots 0 0 0 0 1 1 1 1
  spline S52 degree 3 poles (14.1513, 34.333) (13.8727, 34.1309) (13.3868, 33.8381) (13.0715, 33.6822) knots 0 0 0 0 1 1 1 1
  spline S53 degree 3 poles (13.0715, 33.6822) (11.8711, 33.0889) (10.2509, 33.3985) (9.352, 34.393) knots 0 0 0 0 1 1 1 1
  spline S54 degree 3 poles (9.352, 34.393) (8.4004, 35.4459) (8.1864, 35.6385) (7.9683, 35.6385) knots 0 0 0 0 1 1 1 1
  spline S55 degree 3 poles (7.9683, 35.6385) (7.7171, 35.6385) (7.2977, 35.2383) (6.9738, 34.6891) knots 0 0 0 0 1 1 1 1
  spline S56 degree 3 poles (6.9738, 34.6891) (6.4989, 33.8843) (4.3788, 33.6094) (3.2207, 34.2025) knots 0 0 0 0 1 1 1 1
  spline S57 degree 3 poles (3.2207, 34.2025) (1.9483, 34.8542) (1.3752, 36.0623) (1.9202, 36.9441) knots 0 0 0 0 1 1 1 1
  spline S58 degree 3 poles (1.9202, 36.9441) (2.1572, 37.3277) (2.6853, 37.619) (3.1435, 37.619) knots 0 0 0 0 1 1 1 1
  spline S59 degree 3 poles (3.1435, 37.619) (3.8871, 37.619) (4.3159, 37.943) (4.3159, 38.505) knots 0 0 0 0 1 1 1 1
  spline S60 degree 3 poles (4.3159, 38.505) (4.3159, 39.0685) (4.1681, 39.1932) (3.1927, 39.4522) knots 0 0 0 0 1 1 1 1
  spline S61 degree 3 poles (3.1927, 39.4522) (2.8902, 39.5325) (2.529, 39.6727) (2.39, 39.7638) knots 0 0 0 0 1 1 1 1
  spline S62 degree 3 poles (2.39, 39.7638) (2.0795, 39.9672) (1.7097, 40.7046) (1.7111, 41.1177) knots 0 0 0 0 1 1 1 1
  spline S63 degree 3 poles (1.7111, 41.1177) (1.7137, 41.8847) (2.5286, 42.9734) (3.3605, 43.321) knots 0 0 0 0 1 1 1 1
  spline S64 degree 3 poles (40.3105, 43.3948) (41.3954, 43.901) (42.2636, 43.9539) (43.1464, 43.5675) knots 0 0 0 0 1 1 1 1
  spline S65 degree 3 poles (43.1464, 43.5675) (43.6121, 43.3637) (44.0986, 42.8484) (44.1975, 42.454) knots 0 0 0 0 1 1 1 1
  spline S66 degree 3 poles (44.1975, 42.454) (44.2329, 42.313) (44.2296, 41.9062) (44.1901, 41.55) knots 0 0 0 0 1 1 1 1
  spline S67 degree 3 poles (44.1901, 41.55) (44.0616, 40.3913) (44.0787, 40.2083) (44.3356, 40.0003) knots 0 0 0 0 1 1 1 1
  spline S68 degree 3 poles (44.3356, 40.0003) (44.7112, 39.6961) (45.1086, 39.7683) (46.0893, 40.3188) knots 0 0 0 0 1 1 1 1
  spline S69 degree 3 poles (46.0893, 40.3188) (47.5056, 41.1136) (48.2545, 41.3947) (49.1098, 41.4522) knots 0 0 0 0 1 1 1 1
  spline S70 degree 3 poles (49.1098, 41.4522) (50.0601, 41.5161) (50.6688, 41.3509) (51.2194, 40.8796) knots 0 0 0 0 1 1 1 1
  spline S71 degree 3 poles (51.2194, 40.8796) (51.7463, 40.4286) (51.9622, 40.0221) (51.9699, 39.4669) knots 0 0 0 0 1 1 1 1
  spline S72 degree 3 poles (51.9699, 39.4669) (51.9747, 39.1179) (51.9177, 38.9851) (51.6667, 38.7609) knots 0 0 0 0 1 1 1 1
  spline S73 degree 3 poles (51.6667, 38.7609) (51.4967, 38.6089) (51.1707, 38.4548) (50.9423, 38.4183) knots 0 0 0 0 1 1 1 1
  spline S74 degree 3 poles (50.9423, 38.4183) (50.0539, 38.2762) (49.4995, 37.6121) (49.7804, 37.0264) knots 0 0 0 0 1 1 1 1
  spline S75 degree 3 poles (49.7804, 37.0264) (49.9949, 36.579) (50.335, 36.453) (51.1465, 36.5202) knots 0 0 0 0 1 1 1 1
  spline S76 degree 3 poles (51.1465, 36.5202) (51.7992, 36.5743) (51.8736, 36.5589) (52.1107, 36.3219) knots 0 0 0 0 1 1 1 1
  spline S77 degree 3 poles (52.1107, 36.3219) (52.632, 35.8005) (52.3398, 34.5008) (51.5692, 33.913) knots 0 0 0 0 1 1 1 1
  spline S78 degree 3 poles (51.5692, 33.913) (50.1664, 32.8431) (48.1142, 32.4761) (46.4453, 32.9969) knots 0 0 0 0 1 1 1 1
  spline S79 degree 3 poles (46.4453, 32.9969) (45.8057, 33.1965) (44.9544, 33.904) (44.6602, 34.4802) knots 0 0 0 0 1 1 1 1
  spline S80 degree 3 poles (44.6602, 34.4802) (44.2129, 35.3568) (43.7112, 35.4679) (42.8564, 34.8799) knots 0 0 0 0 1 1 1 1
  spline S81 degree 3 poles (42.8564, 34.8799) (42.5554, 34.6729) (42.0276, 34.3719) (41.6837, 34.2111) knots 0 0 0 0 1 1 1 1
  spline S82 degree 3 poles (41.6837, 34.2111) (41.1075, 33.9417) (40.9598, 33.9187) (39.8075, 33.9187) knots 0 0 0 0 1 1 1 1
  line L8 (39.8075, 33.9187) -> (38.5567, 33.9187)
  line L9 (38.5567, 33.9187) -> (37.6186, 34.4148)
  spline S83 degree 3 poles (37.6186, 34.4148) (37.1026, 34.6877) (36.539, 34.9376) (36.3661, 34.9702) knots 0 0 0 0 1 1 1 1
  spline S84 degree 3 poles (36.3661, 34.9702) (35.922, 35.0539) (35.5337, 34.7143) (35.1462, 33.9031) knots 0 0 0 0 1 1 1 1
  spline S85 degree 3 poles (35.1462, 33.9031) (34.2767, 32.0829) (32.5077, 31.1785) (31.2082, 31.8899) knots 0 0 0 0 1 1 1 1
  spline S86 degree 3 poles (31.2082, 31.8899) (30.5745, 32.2368) (30.2974, 32.7818) (30.4669, 33.3475) knots 0 0 0 0 1 1 1 1
  spline S87 degree 3 poles (30.4669, 33.3475) (30.6161, 33.8457) (31.3598, 34.532) (32.2646, 35.0067) knots 0 0 0 0 1 1 1 1
  spline S88 degree 3 poles (32.2646, 35.0067) (33.1402, 35.466) (33.3971, 35.7096) (33.3971, 36.0805) knots 0 0 0 0 1 1 1 1
  spline S89 degree 3 poles (33.3971, 36.0805) (33.3971, 36.501) (33.238, 36.7542) (32.8468, 36.9565) knots 0 0 0 0 1 1 1 1
  spline S90 degree 3 poles (32.8468, 36.9565) (31.0444, 37.8883) (30.5759, 39.9699) (31.8443, 41.4109) knots 0 0 0 0 1 1 1 1
  spline S91 degree 3 poles (31.8443, 41.4109) (32.3815, 42.0212) (32.9483, 42.3169) (33.7139, 42.3863) knots 0 0 0 0 1 1 1 1
  spline S92 degree 3 poles (33.7139, 42.3863) (34.5937, 42.4661) (35.2523, 42.2098) (36.037, 41.4824) knots 0 0 0 0 1 1 1 1
  spline S93 degree 3 poles (36.037, 41.4824) (36.3909, 41.1543) (36.763, 40.8557) (36.8638, 40.8189) knots 0 0 0 0 1 1 1 1
  spline S94 degree 3 poles (36.8638, 40.8189) (37.192, 40.6989) (37.5089, 40.9167) (38.6147, 42.0227) knots 0 0 0 0 1 1 1 1
  spline S95 degree 3 poles (38.6147, 42.0227) (39.4081, 42.8162) (39.8679, 43.1882) (40.3105, 43.3948) knots 0 0 0 0 1 1 1 1
  spline S96 degree 3 poles (3.8396, 28.1591) (3.6928, 25.8896) (3.7601, 22.8302) (4.0082, 20.7539) knots 0 0 0 0 1 1 1 1
  ellipse E0 centre (58.4946, 46.0269) end of major axis (108.5558, 82.8636) minor radius 37.1858 (4.0082, 20.7539) -> (11.1287, 6.1499) ccw
  spline S97 degree 3 poles (11.1287, 6.1499) (15.8219, 1.7292) (21.8181, -0.6374) (28.7719, -0.8627) knots 0 0 0 0 1 1 1 1
  ellipse E1 centre (5.0131, 40.0097) end of major axis (43.6862, 4.3261) minor radius 27.1643 (28.7719, -0.8627) -> (39.0808, 0.9877) ccw
  spline S98 degree 3 poles (39.0808, 0.9877) (40.5743, 1.6901) (41.6727, 2.4153) (42.7258, 3.4112) knots 0 0 0 0 1 1 1 1
  spline S99 degree 3 poles (42.7258, 3.4112) (44.4016, 4.9959) (45.589, 6.8874) (46.5056, 9.5421) (46.9414, 10.8042) (47.3249, 12.2429) (47.6965, 13.9335) knots 0 0 0 0 0.677783 0.677783 0.677783 1 1 1 1
  spline S100 degree 3 poles (47.6965, 13.9335) (48.7263, 18.6186) (49.1132, 21.8227) (49.3958, 27.9744) knots 0 0 0 0 1 1 1 1
  ellipse E2 centre (49.445, 28.2243) end of major axis (49.5599, 30.6408) minor radius 0.0375 (49.4993, 29.9265) -> (49.3958, 27.9744) ccw
  spline S101 degree 3 poles (49.4993, 29.9265) (51.3935, 30.3328) (52.9435, 31.0564) (54.0116, 32.193) (54.363, 32.5669) (54.6579, 32.9856) (54.882, 33.4409) knots 0.033409 0.033409 0.033409 0.033409 0.760746 0.760746 0.760746 0.999997 0.999997 0.999997 0.999997
  spline S102 degree 3 poles (54.882, 33.4409) (55.0347, 33.7513) (55.1727, 34.0995) (55.2323, 34.4752) (55.2709, 34.7187) (55.2821, 34.9498) (55.2846, 35.2136) knots 0 0 0 0 0.549059 0.549059 0.549059 0.90483 0.90483 0.90483 0.90483
  line L10 (55.2846, 35.2136) -> (55.2832, 35.6451)
  spline S103 degree 3 poles (55.2832, 35.6451) (55.2771, 35.9972) (55.2543, 36.309) (55.1786, 36.6345) (55.1024, 36.9617) (54.9878, 37.2507) (54.8436, 37.5871) knots 0.088946 0.088946 0.088946 0.088946 0.543269 0.543269 0.543269 1 1 1 1
  line L11 (54.8436, 37.5871) -> (54.6708, 37.9902)
  line L12 (54.6708, 37.9902) -> (54.7256, 38.1789)
  spline S104 degree 3 poles (54.7256, 38.1789) (55.1949, 39.793) (54.7298, 41.4712) (53.6604, 42.6498) (52.9721, 43.4084) (52.0402, 43.976) (50.9574, 44.2653) knots 0 0 0 0 0.608426 0.608426 0.608426 1 1 1 1
  spline S105 degree 3 poles (50.9574, 44.2653) (49.8818, 44.5526) (48.7117, 44.4734) (47.3744, 44.1183) (47.178, 44.0661) (46.9771, 44.0079) (46.771, 43.9438) knots 0 0 0 0 0.824545 0.824545 0.824545 0.945665 0.945665 0.945665 0.945665
  spline S106 degree 3 poles (46.771, 43.9438) (46.7093, 44.062) (46.6405, 44.1796) (46.5676, 44.2944) (46.2623, 44.7749) (45.8902, 45.2321) (45.4363, 45.6075) (45.3884, 45.647) (45.3392, 45.6858) (45.2879, 45.7236) knots 0.223295 0.223295 0.223295 0.223295 0.361232 0.361232 0.361232 0.939053 0.939053 0.939053 1 1 1 1
  spline S107 degree 3 poles (45.2879, 45.7236) (44.2745, 46.4714) (42.9911, 46.772) (41.707, 46.737) (41.2318, 46.724) (40.7551, 46.6601) (40.2904, 46.5351) knots 0.000002 0.000002 0.000002 0.000002 0.729882 0.729882 0.729882 1 1 1 1
  spline S108 degree 3 poles (40.2904, 46.5351) (39.1403, 46.2258) (38.0053, 45.5417) (37.0282, 44.651) knots 0.000001 0.000001 0.000001 0.000001 1 1 1 1
  line L13 (37.0282, 44.651) -> (36.9035, 44.5374)
  spline S109 degree 3 poles (36.9035, 44.5374) (35.1678, 45.5188) (33.1775, 45.6076) (31.5191, 44.8193) (30.4628, 44.3172) (29.5504, 43.4745) (28.8905, 42.373) knots 0.019099 0.019099 0.019099 0.019099 0.618328 0.618328 0.618328 1 1 1 1
  spline S110 degree 3 poles (28.8905, 42.373) (28.2356, 41.2799) (28.0251, 39.987) (28.2891, 38.7134) (28.4327, 38.0204) (28.7011, 37.3303) (29.0737, 36.6286) knots 0 0 0 0 0.647645 0.647645 0.647645 1 1 1 1
  line L14 (29.0737, 36.6286) -> (29.1612, 36.4638)
  line L15 (29.1612, 36.4638) -> (28.9908, 36.2914)
  spline S111 degree 3 poles (28.9908, 36.2914) (28.3897, 35.6836) (27.931, 35.0843) (27.6841, 34.3672) (27.522, 33.8963) (27.4651, 33.4076) (27.4689, 32.9193) knots 0 0 0 0 0.603605 0.603605 0.603605 1 1 1 1
  spline S112 degree 3 poles (27.4689, 32.9193) (27.4781, 31.7149) (28.0681, 30.6219) (28.9533, 29.8689) (29.5522, 29.3594) (30.2878, 28.9905) (31.1058, 28.7908) knots 0 0 0 0 0.569109 0.569109 0.569109 0.954182 0.954182 0.954182 0.954182
  ellipse E3 centre (31.0764, 27.6801) end of major axis (31.0429, 29.675) minor radius 0.0578 (31.1352, 27.6181) -> (31.1058, 28.7908) ccw
  spline S113 degree 3 poles (31.1352, 27.6181) (31.1644, 25.7831) (31.0814, 24.7731) (30.8193, 23.7418) (30.754, 23.485) (30.6766, 23.2243) (30.5839, 22.9462) knots 0 0 0 0 0.800641 0.800641 0.800641 1 1 1 1
  spline S114 degree 3 poles (30.5839, 22.9462) (29.9756, 21.1214) (28.9014, 19.8352) (27.6291, 19.2047) knots 0 0 0 0 1 1 1 1
  spline S115 degree 3 poles (27.6291, 19.2047) (26.8945, 18.8407) (26.4461, 18.7298) (25.9454, 18.7349) (25.7421, 18.7369) (25.5228, 18.7611) (25.2651, 18.8137) knots 0 0 0 0 0.711303 0.711303 0.711303 1 1 1 1
  spline S116 degree 3 poles (25.2651, 18.8137) (23.7232, 19.1281) (22.4595, 20.0877) (21.5265, 21.709) (21.0344, 22.5641) (20.647, 23.6026) (20.4034, 24.8024) knots 0 0 0 0 0.654705 0.654705 0.654705 1 1 1 1
  spline S117 degree 3 poles (20.4034, 24.8024) (20.2739, 25.4408) (20.1421, 26.5799) (20.0696, 27.6039) (20.0342, 28.1041) (20.0114, 28.5828) (20.0045, 28.9687) knots 0 0 0 0 0.457255 0.457255 0.457255 0.680586 0.680586 0.680586 0.680586
  ellipse E4 centre (21.8994, 28.801) end of major axis (24.7102, 28.7135) minor radius 0.1473 (20.5728, 28.9721) -> (20.0045, 28.9687) ccw
  spline S118 degree 3 poles (20.5728, 28.9721) (21.4581, 28.9695) (21.9205, 28.9661) (22.3941, 29.0471) (22.71, 29.1012) (22.9935, 29.2034) (23.2325, 29.3044) knots 0 0 0 0 0.599835 0.599835 0.599835 1 1 1 1
  spline S119 degree 3 poles (23.2325, 29.3044) (24.2399, 29.7303) (25.0756, 30.3613) (25.5649, 31.2416) (25.8255, 31.7103) (25.9766, 32.236) (26.0196, 32.7724) knots 0.000002 0.000002 0.000002 0.000002 0.65253 0.65253 0.65253 1 1 1 1
  spline S120 degree 3 poles (26.0196, 32.7724) (26.0464, 33.1056) (26.0575, 33.4303) (25.9898, 33.7774) (25.9304, 34.0819) (25.8237, 34.343) (25.7057, 34.6008) knots 0 0 0 0 0.532706 0.532706 0.532706 1 1 1 1
  ellipse E5 centre (16.0287, 33.8196) end of major axis (26.0555, 32.469) minor radius 5.942 (25.7057, 34.6008) -> (25.0063, 35.7274) ccw
  spline S121 degree 3 poles (25.0063, 35.7274) (25.2152, 36.1653) (25.3445, 36.6528) (25.3876, 37.161) (25.3966, 37.268) (25.4033, 37.3773) (25.4085, 37.4918) knots 0.077995 0.077995 0.077995 0.077995 0.83962 0.83962 0.83962 1 1 1 1
  spline S122 degree 3 poles (25.4085, 37.4918) (25.4258, 37.868) (25.439, 38.1756) (25.3733, 38.5347) (25.3129, 38.8652) (25.1915, 39.151) (25.0593, 39.4265) (25.0387, 39.4695) (25.0174, 39.513) (24.9954, 39.5579) knots 0 0 0 0 0.484601 0.484601 0.484601 0.930484 0.930484 0.930484 1 1 1 1
  spline S123 degree 3 poles (24.9954, 39.5579) (24.5918, 40.3776) (23.9772, 41.085) (23.1648, 41.5103) (22.385, 41.9186) (21.4967, 42.0784) (20.4603, 42.1269) knots 0 0 0 0 0.510228 0.510228 0.510228 1 1 1 1
  line L16 (20.4603, 42.1269) -> (20.1789, 42.1401)
  spline S124 degree 3 poles (20.1789, 42.1401) (19.8683, 42.9655) (19.3311, 43.6836) (18.669, 44.2614) (18.1917, 44.6778) (17.6457, 45.021) (17.0294, 45.2285) knots 0.1236 0.1236 0.1236 0.1236 0.632884 0.632884 0.632884 1 1 1 1
  spline S125 degree 3 poles (17.0294, 45.2285) (15.6679, 45.6868) (14.1945, 45.6326) (12.6935, 45.1125) (12.1298, 44.9172) (11.5566, 44.6602) (10.9624, 44.3448) knots 0 0 0 0 0.726997 0.726997 0.726997 1 1 1 1
  spline S126 degree 3 poles (10.9624, 44.3448) (10.8083, 44.263) (10.6793, 44.1929) (10.573, 44.1362) knots 0 0 0 0 0.122244 0.122244 0.122244 0.122244
  spline S127 degree 3 poles (10.573, 44.1362) (10.4946, 44.2052) (10.4022, 44.2872) (10.2936, 44.382) knots 0.893888 0.893888 0.893888 0.893888 1 1 1 1
  ellipse E6 centre (-1.4228, 24.3555) end of major axis (-10.8734, 2.8827) minor radius 14.2538 (10.2936, 44.382) -> (7.2449, 46.1286) ccw
  spline S128 degree 3 poles (7.2449, 46.1286) (6.4114, 46.403) (5.4613, 46.5014) (4.5483, 46.4889) (3.8849, 46.4798) (3.2641, 46.4203) (2.6738, 46.2166) knots 0.000001 0.000001 0.000001 0.000001 0.579134 0.579134 0.579134 1 1 1 1
  spline S129 degree 3 poles (2.6737, 46.2166) (0.624, 45.5094) (-0.7902, 43.8549) (-1.106, 41.9528) (-1.287, 40.8624) (-1.1003, 39.6959) (-0.5192, 38.6497) knots 0 0 0 0 0.618555 0.618555 0.618555 0.973163 0.973163 0.973163 0.973163
  spline S130 degree 3 poles (-0.5192, 38.6497) (-0.9554, 37.9197) (-1.2418, 37.1573) (-1.2576, 36.3503) (-1.2716, 35.6348) (-1.0747, 34.9439) (-0.7598, 34.2709) knots 0.006673 0.006673 0.006673 0.006673 0.533212 0.533212 0.533212 1 1 1 1
  spline S131 degree 3 poles (-0.7598, 34.2709) (0.1145, 32.4027) (1.9335, 31.179) (4.0147, 30.9406) knots 0 0 0 0 0.893312 0.893312 0.893312 0.893312
  spline S132 degree 3 poles (4.0147, 30.9406) (3.9761, 30.3012) (3.9008, 29.105) (3.8396, 28.1591) knots 0.081568 0.081568 0.081568 0.081568 1 1 1 1
  spline S133 degree 3 poles (29.7007, 2.1311) (29.5989, 2.131) (29.4934, 2.1308) (29.3841, 2.1308) knots 0.955909 0.955909 0.955909 0.955909 1 1 1 1
  spline S134 degree 3 poles (29.3841, 2.1308) (26.2893, 2.1292) (25.7344, 2.1938) (23.1155, 2.861) knots 0 0 0 0 1 1 1 1
  spline S135 degree 3 poles (23.1155, 2.861) (15.8271, 4.7179) (10.0738, 9.8891) (7.9282, 16.5117) knots 0 0 0 0 1 1 1 1
  spline S136 degree 3 poles (7.9282, 16.5117) (7.4178, 18.087) (7.2808, 18.6726) (7.0133, 20.4204) knots 0 0 0 0 1 1 1 1
  spline S137 degree 3 poles (7.0133, 20.4204) (6.814, 21.7234) (6.7809, 22.3775) (6.7737, 25.1631) knots 0 0 0 0 1 1 1 1
  spline S138 degree 3 poles (6.7737, 25.1631) (6.7643, 28.8189) (6.9545, 31.8997) (7.2227, 32.4341) knots 0 0 0 0 1 1 1 1
  spline S139 degree 3 poles (7.2227, 32.4341) (7.3731, 32.7338) (7.7563, 33.027) (8.0031, 33.0312) knots 0 0 0 0 1 1 1 1
  spline S140 degree 3 poles (8.0031, 33.0312) (8.0532, 33.032) (8.369, 32.8492) (8.705, 32.6248) knots 0 0 0 0 1 1 1 1
  spline S141 degree 3 poles (8.705, 32.6248) (9.2851, 32.2374) (9.8665, 32.0076) (11.2214, 31.6303) knots 0 0 0 0 1 1 1 1
  spline S142 degree 3 poles (11.2214, 31.6303) (11.8742, 31.4485) (11.8914, 31.4155) (11.7143, 30.6874) knots 0 0 0 0 1 1 1 1
  spline S143 degree 3 poles (11.7143, 30.6874) (10.9845, 27.6875) (10.9096, 23.7891) (11.5242, 20.7853) knots 0 0 0 0 1 1 1 1
  spline S144 degree 3 poles (11.5242, 20.7853) (12.8947, 14.087) (17.7674, 9.0084) (23.8364, 7.9527) knots 0 0 0 0 1 1 1 1
  spline S145 degree 3 poles (23.8364, 7.9527) (24.5674, 7.8255) (25.2101, 7.7982) (26.5177, 7.8388) knots 0 0 0 0 1 1 1 1